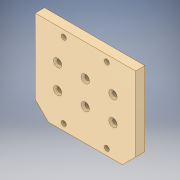
# Autodesk Inventor part: DPLX_P032_VIPE Insulation Middle
Saved by Autodesk Inventor 2018 (Build 220112000, 112)
## iProperties
Created: 2017-12-19
Part Number: DPLX_P032_VIPE Insulation Middle
Material: Polyethylene, High Density
Document SubType Name: Modeling
Designer: Sam
Density: 0.952 g/cm^3
Appearance: Smooth - Off-White
Mass: 23.4327 g
Surface Area: 99.1997 cm^2
Volume: 24.6142 cm^3
Author: Sam
Comments: http://www.eplastics.com/Plastic/G9-G10-FR4-glass-epoxy-sheet/G10NAT-250X12X12
Autodesk Inventor part; units mm, degrees
ref_plane "YZ Plane" through (0, 0, 0) normal (1, 0, 0) x (0, 1, 0)
ref_plane "XZ Plane" through (0, 0, 0) normal (0, 1, 0) x (-1, 0, 0)
ref_plane "XY Plane" through (0, 0, 0) normal (0, 0, 1) x (1, 0, 0)
sketch "Sketch1" plane through (0, 0, 0) normal (0, 0, 1) x (1, 0, 0)
  line L0 (-34.036, -29.7688) -> (34.036, -29.7688)
  line L1 (34.036, -29.7688) -> (34.036, 29.7688)
  line L2 (34.036, 29.7688) -> (-34.036, 29.7688)
  line L3 (-34.036, 29.7688) -> (-34.036, -29.7688)
  line L4 (-34.036, -29.7688) -> (34.036, 29.7688) construction
  line L5 (34.036, -29.7688) -> (-34.036, 29.7688) construction
  point P0 (0, 0)
  dimension "d0" = 68.072
  dimension "d1" = 59.5376
  constraints: 12 end point, 2 midpoint, 2 parallel, 1 horizontal, 1 perpendicular
  measures "d0" distance of L2.end L1.end
  measures "d1" distance of L1.end L0.end
extrude "Extrusion1" add sketch "Sketch1" along normal blind 6.35
sketch "Sketch3" plane through (0, 0, 6.35) normal (0, 0, 1) x (1, 0, 0)
  line L0 (34.036, 29.7688) -> (-34.036, 29.7688) projected
  line L1 (-34.036, -29.7688) -> (34.036, -29.7688) projected
  line L2 (-34.036, 29.7688) -> (-34.036, -29.7688) projected
  line L3 (34.036, -29.7688) -> (34.036, 29.7688) projected
  point P0 (0, 0)
  point P1 (-18.796, 8.1788)
  point P2 (-18.796, -8.1788)
  point P3 (18.796, -8.1788)
  point P4 (18.796, 8.1788)
  point P5 (0, 8.1788)
  point P6 (0, -8.1788)
  dimension "d17" = 21.59
  dimension "d18" = 21.59
  dimension "d19" = 15.24
  dimension "d20" = 15.24
  dimension "d21" = 18.796
  dimension "d23" = 37.592
  constraints: 4 horizontal alignment, 3 vertical alignment
  measures "d17" distance from line of L0 point (-18.796, 8.179)
  measures "d18" distance from line of point (-18.796, -8.179) L1
  measures "d19" distance from line of L2 point (-18.796, 8.179)
  measures "d20" distance from line of L3 point (18.796, 8.179)
  measures "d21" distance of point (0, 8.179) point (-18.796, 8.179)
  measures "d23" distance of point (18.796, 8.179) point (-18.796, 8.179)
hole "Hole2" at (-18.796, 8.1788, 6.35) at (-18.796, -8.1788, 6.35) at (18.796, -8.1788, 6.35) at (18.796, 8.1788, 6.35) at (0, 8.1788, 6.35) at (0, -8.1788, 6.35) direction (0, 0, -1) diameter 3 depth 25.4 tip angle 118 countersink diameter 5.6 countersink angle 90
chamfer "Chamfer1" distance 8.89 angle 45 2 edges at (-34.036, -29.7688, 3.175) (34.036, -29.7688, 3.175)
sketch "Sketch4" plane through (0, 0, 0) normal (0, 0, -1) x (-1, 0, 0)
  circle A0 centre (-14.605, -25.4024) radius 1.7018 projected
  circle A1 centre (14.605, -25.4024) radius 1.7018 projected
  circle A2 centre (14.605, 25.3976) radius 1.7018 projected
  circle A3 centre (-14.605, 25.3976) radius 1.7018 projected
  point P0 (0, 0)
hole "Hole3" at (14.605, -25.4024, 0) at (-14.605, -25.4024, 0) at (-14.605, 25.3976, 0) at (14.605, 25.3976, 0) direction (0, 0, 1) diameter 3.4036 end through all countersink diameter 6.2992 countersink angle 90 clearance for "Flat Head Machine Screw" size "M3" standard "Ansi Metric M Profile"
equation "\"d18\" = d17"
equation "\"d20\" = d19"
equation "\"d21\" = 0.5 * d23"
body "Solid1"
